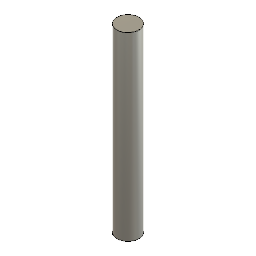
Robot_CDFR_2022 v8 (Autodesk Fusion 360 archive; units mm, degrees)
design "Barre_Odometry"
Autodesk Fusion 360 part; units mm, degrees
sketch "Sketch1" plane through (0, 0, 0) normal (0, 1, 0) x (1, 0, 0)
  circle A0 centre (0, 0) radius 4
  dimension "d1" = 8
  measures "d1" diameter of A0
extrude "Extrude1" add sketch "Sketch1" along normal blind 65

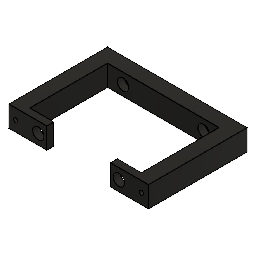
design "Barre_Odometry"
Autodesk Fusion 360 part; units mm, degrees
sketch "Sketch1" plane through (0, 0, 0) normal (0, 1, 0) x (1, 0, 0)
  line L0 (0, 0) -> (99, 0)
  line L1 (99, 0) -> (99, -70)
  line L2 (0, -70) -> (0, 0)
  line L3 (0, -70) -> (27, -70)
  line L4 (99, -70) -> (72, -70)
  line L5 (72, -70) -> (72, -65)
  line L6 (27, -70) -> (27, -65)
  line L7 (27, -65) -> (10, -65)
  line L8 (72, -65) -> (89, -65)
  line L9 (10, -65) -> (10, -10)
  line L10 (89, -65) -> (89, -10)
  line L11 (10, -10) -> (89, -10)
  dimension "d1" = 70
  dimension "d2" = 99
  dimension "d3" = 27
  dimension "d5" = 5
  dimension "d6" = 17
  dimension "d7" = 10
  measures "d1" distance of L0.start
  measures "d3" distance of L0.start
  measures "d6" distance of L0.start
  measures "d7" distance of L0.start
extrude "Extrude1" add sketch "Sketch1" along normal blind 15
sketch "Sketch2" plane through (0, 0, 0) normal (0, 0, -1) x (-1, 0, 0)
  line L0 (-99, 0) -> (0, 0)
  line L1 (0, 0) -> (0, 15)
  line L2 (0, 15) -> (-99, 15)
  line L3 (-99, 15) -> (-99, 0)
  circle A0 centre (-94, 7.5) radius 1.5
  circle A1 centre (-5, 7.5) radius 1.5
  dimension "d10" = 3
  dimension "d11" = 5
  dimension "d12" = 5
  measures "d10" diameter of A1
  measures "d11" distance of L0.end
  measures "d12" distance of L0.end
extrude "Extrude2" cut sketch "Sketch2" against normal up to surface (70 mm away) contours A0 | A1
sketch "Sketch4" plane through (0, 0, 10) normal (0, 0, 1) x (1, 0, 0)
  line L0 (10, 0) -> (89, 0)
  line L1 (89, 0) -> (89, 15)
  line L2 (89, 15) -> (10, 15)
  line L3 (10, 15) -> (10, 0)
  circle A0 centre (21, 7.4297) radius 4
  circle A1 centre (78, 7.4297) radius 4
  dimension "d15" = 8
  dimension "d16" = 57
  dimension "d17" = 11
  measures "d15" diameter of A0
extrude "Extrude3" cut sketch "Sketch4" along normal up to surface (60 mm away) and the other way blind 5 contours A0 | A1
equation "d17 = ( ( 79 - 57 ) / 2 ) * 1 mm"

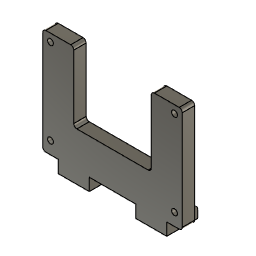
design "Support PCB"
Autodesk Fusion 360 part; units mm, degrees
sketch "Esquisse1" plane through (0, 0, 0) normal (0, 1, 0) x (1, 0, 0)
  line L0 (0, 0) -> (90, 0)
  line L1 (90, 0) -> (90, -68)
  line L2 (90, -68) -> (0, -68)
  line L3 (0, -68) -> (0, 0)
  circle A0 centre (5, -63) radius 1.9
  circle A1 centre (85, -63) radius 1.9
  circle A2 centre (85, -8) radius 1.9
  circle A3 centre (5, -8) radius 1.9
  line L4 (20, -68) -> (20, -23)
  line L5 (20, -23) -> (70, -23)
  line L6 (70, -23) -> (70, -68)
  line L7 (10, 0) -> (30, 0)
  line L8 (30, 0) -> (30, 8)
  line L9 (30, 8) -> (10, 8)
  line L10 (10, 8) -> (10, 0)
  line L11 (80, 0) -> (60, 0)
  line L12 (60, 0) -> (60, 8)
  line L13 (60, 8) -> (80, 8)
  line L14 (80, 8) -> (80, 0)
  dimension "d4" = 68
  dimension "d5" = 90
  dimension "d6" = 3.8
  dimension "d7" = 5
  dimension "d8" = 5
  dimension "d9" = 3.8
  dimension "d10" = 3.8
  dimension "d11" = 3.8
  dimension "d12" = 8
  dimension "d13" = 5
  dimension "d14" = 8
  dimension "d15" = 5
  dimension "d16" = 5
  dimension "d17" = 5
  dimension "d18" = 45
  dimension "d19" = 20
  dimension "d20" = 20
  dimension "d22" = 10
  dimension "d23" = 8
  dimension "d24" = 10
  dimension "d25" = 8
  dimension "d26" = 20
  dimension "d27" = 20
  constraint horizontal L0
  constraint vertical L1
  constraint horizontal L2
  constraint vertical L3
  constraint coincident L0.start L3.end
  constraint coincident L2 L4.start
  constraint perpendicular L2 L4
  constraint perpendicular L4 L5
  constraint coincident L2 L6.end
  constraint perpendicular L2 L6
  constraint horizontal L7
  constraint vertical L8
  constraint horizontal L9
  constraint vertical L10
  constraint coincident L0 L7.start
  constraint horizontal L11
  constraint vertical L12
  constraint horizontal L13
  constraint vertical L14
  constraint coincident L0 L11.start
  measures "d4" distance of L0.start L2.end
  measures "d5" distance of L1.end L2.end
  measures "d6" diameter of A0
  measures "d7" distance of L2 A0.centre
  measures "d8" distance of L3 A0.centre
  measures "d9" diameter of A1
  measures "d10" diameter of A2
  measures "d11" diameter of A3
  measures "d12" distance of L0 A3.centre
  measures "d13" distance of L3 A3.centre
  measures "d14" distance of L0 A2.centre
  measures "d15" distance of L1 A2.centre
  measures "d16" distance of L2 A1.centre
  measures "d17" distance of L1 A1.centre
  measures "d18" distance of L4.start L4.end
  measures "d19" distance of L3 L4
  measures "d20" distance of L1 L6
  measures "d22" distance of L3 L10
  measures "d23" distance of L7.start L9.end
  measures "d24" distance of L1 L14
  measures "d25" distance of L11.start L13.end
  measures "d26" distance of L8.end L9.end
  measures "d27" distance of L12.end L13.end
extrude "Extrusion1" add sketch "Esquisse1" along normal blind 8 contours L0 L1 L2 L3 L4 L5 L6 L7 L11
extrude "Extrusion2" add sketch "Esquisse1" along normal blind 20 contours L0 L7 L8 L9 L10
extrude "Extrusion3" add sketch "Esquisse1" along normal blind 20 contours L0 L11 L12 L13 L14
sketch "Esquisse2" plane through (0, 0, 0) normal (0, 0, 1) x (1, 0, 0)
sketch "Esquisse3" plane through (0, 0, 0) normal (0, 0, 1) x (-1, 0, 0)
  line L0 (-10, -8) -> (-30, -8)
  line L1 (-30, -8) -> (-30, -20)
  line L2 (-30, -20) -> (-10, -20)
  line L3 (-10, -20) -> (-10, -8)
  circle A0 centre (-16, -13) radius 2.1
  circle A1 centre (-74, -13) radius 2.1
  dimension "d34" = 4.2
  dimension "d35" = 4.2
  dimension "d36" = 58
  dimension "d37" = 6
  dimension "d38" = 7
  dimension "d41" = 7
  measures "d34" diameter of A0
  measures "d35" diameter of A1
  measures "d36" horizontal distance of A0.centre A1.centre
  measures "d37" distance of L3 A0.centre
  measures "d38" distance of L2 A0.centre
  measures "d41" distance of L2 A1.centre
extrude "Extrusion4" cut sketch "Esquisse3" against normal blind 8 contours A0 | A1
fillet "Congé1" radius 3 1 edges at (70, 20, 0)
fillet "Congé2" radius 3 1 edges at (20, 20, 0)
fillet "Congé3" radius 2 1 edges at (70, 4, 68)
fillet "Congé4" radius 2 1 edges at (0, 4, 68)
fillet "Congé5" radius 2 1 edges at (90, 4, 68)
fillet "Congé6" radius 2 1 edges at (20, 4, 68)
fillet "Congé7" radius 2 1 edges at (90, 4, 0)
fillet "Congé8" radius 2 1 edges at (0, 4, 0)
fillet "Congé9" radius 2 1 edges at (70, 4, 23)
fillet "Congé10" radius 2 1 edges at (20, 4, 23)

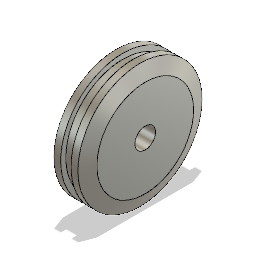
design "Roue_Odometry"
Autodesk Fusion 360 part; units mm, degrees
sketch "Sketch1" plane through (0, 0, 0) normal (0, 1, 0) x (1, 0, 0)
  line L0 (0, 0) -> (10, 0)
  line L1 (5, 0) -> (5, 20.4446) construction
  line L2 (0, 0) -> (0, 14)
  line L3 (0, 14) -> (1.5, 18)
  line L4 (1.5, 18) -> (3.5, 18)
  line L5 (3.5, 18) -> (3.5, 16.5)
  line L6 (3.5, 16.5) -> (6.5, 16.5)
  line L7 (10, 0) -> (10, 14)
  line L8 (6.5, 16.5) -> (6.5, 18)
  line L9 (6.5, 18) -> (8.5, 18)
  line L10 (8.5, 18) -> (10, 14)
  dimension "d1" = 10
  dimension "d2" = 14
  dimension "d3" = 18
  dimension "d4" = 2
  dimension "d5" = 3
  dimension "d6" = 1.5
  measures "d1" distance of L0.start
  measures "d2" distance of L0.start
  measures "d3" distance of L0.start
revolve "Revolve1" add sketch "Sketch1" angle 360 about axis through (0, 0, 0) along (1, 0, 0)
sketch "Sketch2" plane through (10, 0, 0) normal (1, 0, 0) x (0, 0, -1)
  circle A0 centre (0, 0) radius 14
  circle A1 centre (0, 0) radius 3
  dimension "d8" = 6
  measures "d8" diameter of A1
extrude "Extrude1" cut sketch "Sketch2" against normal up to surface (10 mm away) contours A1

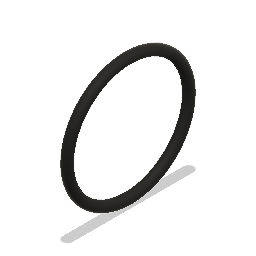
design "Joint_Odometry"
Autodesk Fusion 360 part; units mm, degrees
sketch "Sketch1" plane through (0, 0, 0) normal (0, 1, 0) x (1, 0, 0)
  circle A0 centre (0, 18) radius 1.5
  dimension "d1" = 18
  dimension "d2" = 3
  measures "d1" distance of origin
  measures "d2" diameter of A0
revolve "Revolve1" add sketch "Sketch1" angle 360 about axis through (1.75, 0, 0) along (1, 0, 0)
